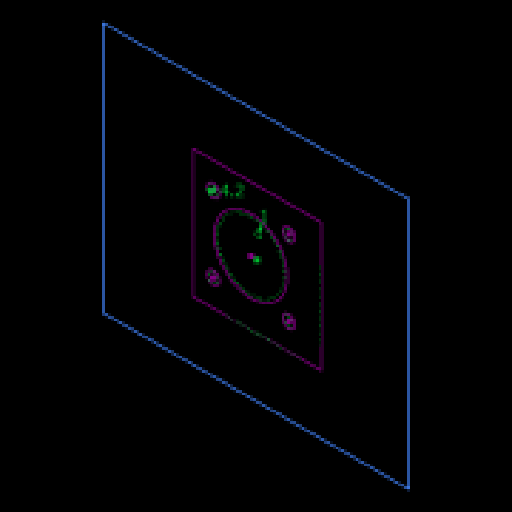
# Autodesk Inventor part: ShoulderEncoderDrillGuide
Saved by Autodesk Inventor 2025.2 (Build 292293000, 293)
## iProperties
Created: 2026-06-27
Part Number: ShoulderEncoderDrillGuide
Material: Generic
Document SubType Name: Modeling
Designer: valer
Density: 1 g/cm^3
Appearance: Default
Author: valer
Autodesk Inventor part; units mm, degrees
ref_plane "YZ Plane" through (0, 0, 0) normal (1, 0, 0) x (0, 1, 0)
ref_plane "XZ Plane" through (0, 0, 0) normal (0, 1, 0) x (-1, 0, 0)
ref_plane "XY Plane" through (0, 0, 0) normal (0, 0, 1) x (1, 0, 0)
sketch "Sketch1" plane through (0, 0, 0) normal (0, 0, 1) x (1, 0, 0)
  line L0 (-21, 20) -> (-21, -20) construction
  line L1 (14.2964, 21) -> (-14.2964, 21) construction
  line L2 (21, -20) -> (21, 20) construction
  line L3 (-14.2964, -21) -> (14.2964, -21) construction
  circle A0 centre (-14.3744, 12.3744) radius 1.621 construction
  circle A1 centre (10.3746, 12.3744) radius 1.621 construction
  circle A2 centre (10.3746, -12.3746) radius 1.621 construction
  circle A3 centre (-14.3744, -12.3746) radius 1.621 construction
  line L4 (-21, 21) -> (21, 21)
  line L5 (21, 21) -> (21, -21)
  line L6 (21, -21) -> (-21, -21)
  line L7 (-21, -21) -> (-21, 21)
  circle A4 centre (-14.3744, 12.3744) radius 2.1
  circle A5 centre (10.3746, 12.3744) radius 2.1
  circle A6 centre (10.3746, -12.3746) radius 2.1
  circle A7 centre (-14.3744, -12.3746) radius 2.1
  circle A8 centre (-2, 0) radius 11 construction
  circle A9 centre (-2, 0) radius 12
  point P0 (0, 0)
  dimension "d0" = 4.2
  dimension "d1" = 1
  constraints: 8 end point, 5 centre point, 5 coincident, 4 collinear, 3 equal radius, 2 parallel, 1 horizontal, 1 perpendicular
  measures "d0" diameter of A4
  measures "d1" radial gap between concentric circles of A9 A8
extrude "Extrusion1" add sketch "Sketch1" along normal blind 5
sketch "Sketch2" plane through (0, 0, 5) normal (0, 0, 1) x (1, 0, 0)
  line L0 (-21, -21) -> (21, -21) projected
  line L1 (21, 21) -> (-21, 21) projected
  line L2 (-21, 21) -> (-21, -21) projected
  line L3 (21, -21) -> (21, -25)
  line L4 (21, -25) -> (-25, -25)
  line L5 (-25, -25) -> (-25, 25)
  line L6 (-25, 25) -> (21, 25)
  line L7 (21, 25) -> (21, 21)
  point P0 (0, 0)
  dimension "d4" = 4
  dimension "d5" = 4
  dimension "d6" = 4
  constraints: 10 end point, 5 perpendicular
  measures "d4" distance between parallel lines of L5 L2
  measures "d5" distance between parallel lines of L4 L0
  measures "d6" distance between parallel lines of L6 L1
extrude "Extrusion2" add sketch "Sketch2" against normal blind 10
fillet "Fillet1" radius 4 2 edges at (-25, -25, 0) (-25, 25, 0)
body "Solid1"
